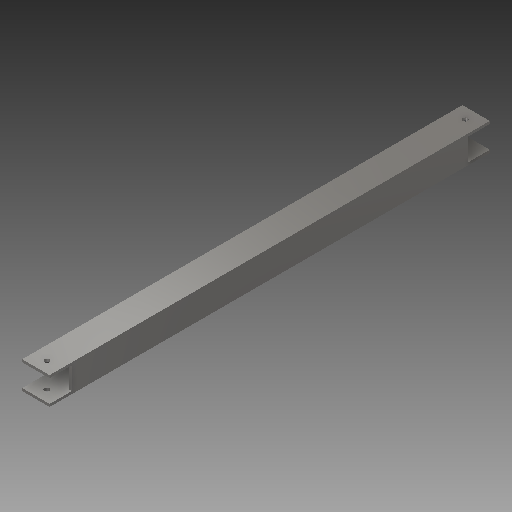
# Autodesk Inventor part: 32in2.0Sq
Saved by Autodesk Inventor 2018 (Build 220112000, 112)
## iProperties
Created: 2018-08-05
Part Number: 32in2.0Sq
Material: Steel, Mild
Document SubType Name: Modeling
Designer: Cole Tucker
Density: 7.85 g/cm^3
Appearance: Semi-Polished
Mass: 5330.35 g
Surface Area: 2890.52 cm^2
Volume: 679.026 cm^3
Author: Cole Tucker
Autodesk Inventor part; units mm, degrees
ref_plane "YZ Plane" through (0, 0, 0) normal (1, 0, 0) x (0, 1, 0)
ref_plane "XZ Plane" through (0, 0, 0) normal (0, 1, 0) x (-1, 0, 0)
ref_plane "XY Plane" through (0, 0, 0) normal (0, 0, 1) x (1, 0, 0)
sketch "Sketch1" plane through (0, 0, 0) normal (0, 0, 1) x (1, 0, 0)
  line L0 (0, 0) -> (50.8, 0)
  line L1 (50.8, 0) -> (50.8, 50.8)
  line L2 (50.8, 50.8) -> (0, 50.8)
  line L3 (0, 50.8) -> (0, 0)
  line L4 (0, 0) -> (4.7625, 0) construction
  line L5 (4.7625, 0) -> (4.7625, 4.7625) construction
  line L6 (4.7625, 4.7625) -> (0, 4.7625) construction
  line L7 (0, 4.7625) -> (0, 0) construction
  line L8 (50.8, 50.8) -> (46.0375, 50.8) construction
  line L9 (46.0375, 50.8) -> (46.0375, 46.0375) construction
  line L10 (46.0375, 46.0375) -> (50.8, 46.0375) construction
  line L11 (50.8, 46.0375) -> (50.8, 50.8) construction
  line L12 (46.0375, 46.0375) -> (4.7625, 46.0375)
  line L13 (4.7625, 46.0375) -> (4.7625, 4.7625)
  line L14 (4.7625, 4.7625) -> (46.0375, 4.7625)
  line L15 (46.0375, 4.7625) -> (46.0375, 46.0375)
  dimension "d0" = 50.8
  dimension "d1" = 50.8
  dimension "d2" = 4.7625
  dimension "d3" = 4.7625
  dimension "d4" = 4.7625
  dimension "d5" = 4.7625
  constraints: 32 end point, 8 parallel, 4 horizontal, 4 perpendicular
  measures "d0" distance of L2.end L1.end
  measures "d1" distance of L1.end L0.end
  measures "d2" distance of L6.end L5.end
  measures "d3" distance of L5.end L4.end
  measures "d4" distance of L10.end L9.end
  measures "d5" distance of L9.end L8.end
extrude "Extrusion1" add sketch "Sketch1" along normal blind 812.8
sketch "Sketch2" plane through (50.8, 0, 0) normal (1, 0, 0) x (0, 0, -1)
  line L0 (0, 4.7625) -> (-812.8, 4.7625) projected
  line L1 (0, 46.0375) -> (-812.8, 46.0375) projected
  line L2 (0, 4.7625) -> (-41.275, 4.7625)
  line L3 (-41.275, 4.7625) -> (-41.275, 46.0375)
  line L4 (-41.275, 46.0375) -> (0, 46.0375)
  line L5 (0, 46.0375) -> (0, 4.7625)
  line L6 (-812.8, 4.7625) -> (-812.8, 46.0375) projected
  line L7 (-812.8, 4.7625) -> (-771.525, 4.7625)
  line L8 (-771.525, 4.7625) -> (-771.525, 46.0375)
  line L9 (-771.525, 46.0375) -> (-812.8, 46.0375)
  line L10 (-812.8, 46.0375) -> (-812.8, 4.7625)
  point P0 (0, 0)
  dimension "d8" = 41.275
  dimension "d9" = 41.275
  constraints: 16 end point, 4 parallel, 2 horizontal, 2 perpendicular, 2 point on line
  measures "d8" distance of L3.end L4.end
  measures "d9" distance of L9.end L8.end
extrude "Extrusion2" cut sketch "Sketch2" against normal blind 50.8 contours L0 L3 L1 L5 | L0 L6 L1 L8
sketch "Sketch3" plane through (0, 0, 0) normal (0, -1, 0) x (1, 0, 0)
  line L0 (46.0375, 41.275) -> (46.0375, 771.525) projected
  line L1 (4.7625, 41.275) -> (0, 41.275) projected
  line L2 (46.0375, 41.275) -> (4.7625, 41.275)
  line L3 (25.4, 41.275) -> (25.4, 0)
  line L4 (50.8, 771.525) -> (46.0375, 771.525) projected
  line L5 (4.7625, 771.525) -> (0, 771.525) projected
  line L6 (46.0375, 771.525) -> (4.7625, 771.525)
  line L7 (25.4, 771.525) -> (25.4, 812.8)
  line L8 (0, 812.8) -> (50.8, 812.8) projected
  point P0 (0, 0)
  point P1 (25.4, 20.6375)
  point P2 (25.4, 792.1625)
  constraints: 8 end point, 5 midpoint, 2 collinear, 1 vertical
hole "Hole1" at (25.4, 0, 20.6375) at (25.4, 0, 792.1625) direction (0, 1, 0) diameter 9.525 depth 50.8 tip angle 118
equation "\"d0\" = d1"
equation "\"d2\" = d3"
equation "\"d4\" = d3"
equation "\"d5\" = d3"
body "Solid1"
